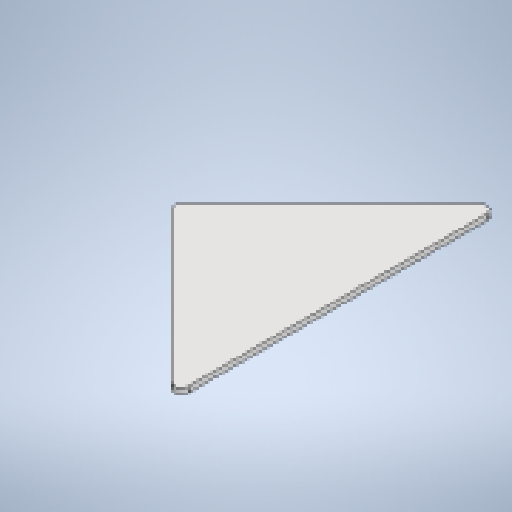
# Autodesk Inventor part: DS-B-503 CAP
Saved by Autodesk Inventor 2025 (Build 290162010, 162A)
## iProperties
Created: 2025-01-16
Part Number: DS-B-503 CAP
Material: Stainless Steel
Document SubType Name: Sheet Metal
Designer: pokla
Density: 8 g/cm^3
Sheet Metal Rule: AISI304 2mm Die16
Appearance: Default
Flat Pattern Width: 2.25858 cm
Flat Pattern Length: 4.31716 cm
Flat Pattern Area: 9.75064 cm^2
Sheet Metal Width: 22.586 mm
Sheet Metal Length: 43.172 mm
Sheet Metal Area: 975.064 mm^2
Author: pokla
Autodesk Inventor part; units mm, degrees
ref_plane "YZ Plane" through (0, 0, 0) normal (1, 0, 0) x (0, 1, 0)
ref_plane "XZ Plane" through (0, 0, 0) normal (0, 1, 0) x (-1, 0, 0)
ref_plane "XY Plane" through (0, 0, 0) normal (0, 0, 1) x (1, 0, 0)
sketch "Sketch1" plane through (0, 0, 0) normal (0, 0, 1) x (1, 0, 0)
  line L0 (0, -23) -> (0, 23)
  line L1 (0, -23) -> (-23, 0)
  line L2 (-23, 0) -> (0, 23)
  point P0 (0, 0)
  point P1 (0, 0)
  point P2 (0, 0)
  dimension "d1" = 46
  dimension "d9" = 23
  measures "d1" distance of L0.start L0.end
  measures "d9" distance from line of L0 L1.end
extrude "Plate1" add sketch "Sketch1" along normal blind 0.8
fillet "Corner Round2" radius 1 3 edges at (0, -23, 0.4) (-23, 0, 0.4) (0, 23, 0.4)
equation "\"d2\" = Thickness"
equation "\"BendReliefWidth\" = Thickness"
equation "\"BendReliefDepth\" = 0.5 * Thickness"
equation "\"CornerReliefSize\" = 4 * Thickness"
equation "\"MinimumRemnant\" = 2 * Thickness"
equation "\"TransitionRadius\" = BendRadius"
equation "\"JacobiRadiusSize\" = BendRadius"
equation "\"GapSize\" = Thickness"
equation "\"Thickness\" = 0.8"
equation "\"BendRadius\" = 2.75"
body "Solid1"
